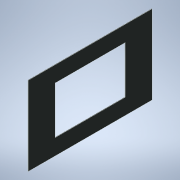
# Autodesk Inventor part: Pieza3
Saved by Autodesk Inventor 2021 (Build 250183000, 183)
## iProperties
Created: 2022-08-16
Part Number: Pieza3
Material: Genérico
Document SubType Name: Modeling
Designer: arthu
Density: 1 g/cm^3
Appearance: Gris plomo - Pulido
Author: arthu
Autodesk Inventor part; units mm, degrees
ref_plane "YZ Plane" through (0, 0, 0) normal (1, 0, 0) x (0, 1, 0)
ref_plane "XZ Plane" through (0, 0, 0) normal (0, 1, 0) x (-1, 0, 0)
ref_plane "XY Plane" through (0, 0, 0) normal (0, 0, 1) x (1, 0, 0)
sketch "Boceto1" plane through (0, 0, 0) normal (1, 0, 0) x (0, 1, 0)
  line L0 (-175, -275) -> (175, -275)
  line L1 (175, -275) -> (175, 275)
  line L2 (175, 275) -> (-175, 275)
  line L3 (-175, 275) -> (-175, -275)
  line L4 (-175, -275) -> (175, 275) construction
  line L5 (175, -275) -> (-175, 275) construction
  line L6 (-105, -155) -> (105, -155)
  line L7 (105, -155) -> (105, 155)
  line L8 (105, 155) -> (-105, 155)
  line L9 (-105, 155) -> (-105, -155)
  line L10 (-105, -155) -> (105, 155) construction
  line L11 (105, -155) -> (-105, 155) construction
  point P0 (0, 0)
  dimension "d0" = 350
  dimension "d1" = 550
  dimension "d2" = 210
  dimension "d3" = 310
  constraints: 24 end point, 4 midpoint, 4 parallel, 2 horizontal, 2 perpendicular
  measures "d0" distance of L2.end L1.end
  measures "d1" distance of L1.end L0.end
  measures "d2" distance of L8.end L7.end
  measures "d3" distance of L7.end L6.end
extrude "Extrusión1" add sketch "Boceto1" along normal blind 2
